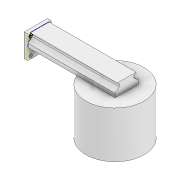
# Autodesk Inventor part: TopBracket
Saved by Autodesk Inventor 2021.1 (Build 251245010, 245A)
## iProperties
Created: 2023-07-02
Part Number: TopBracket
Material: ABS Plastic
Document SubType Name: Modeling
Designer: Drake
Density: 1.06 g/cm^3
Appearance: Smooth - White
Author: Drake
Autodesk Inventor part; units mm, degrees
ref_plane "YZ Plane" through (0, 0, 0) normal (1, 0, 0) x (0, 1, 0)
ref_plane "XZ Plane" through (0, 0, 0) normal (0, 1, 0) x (-1, 0, 0)
sketch "Sketch1" plane through (0, 0, 0) normal (1, 0, 0) x (0, 1, 0)
  line L0 (-20, 20) -> (20, 20)
  line L1 (20, 20) -> (20, -20)
  line L2 (20, -20) -> (-20, -20)
  line L3 (-20, -20) -> (-20, 20)
  line L4 (-20, 20) -> (20, -20) construction
  line L5 (20, 20) -> (-20, -20) construction
  point P0 (0, 0)
  dimension "d0" = 40
  dimension "d1" = 40
  constraints: 12 end point, 2 midpoint, 2 parallel, 1 horizontal, 1 perpendicular
  measures "d0" distance of L1.end L2.end
  measures "d1" distance of L0.end L1.end
extrude "Extrusion1" add sketch "Sketch1" along normal mid plane 6
sketch "Sketch2" plane through (3, 0, 0) normal (1, 0, 0) x (0, 0, -1)
  line L0 (20, 20) -> (-20, 20) projected
  line L1 (-20, 20) -> (-15, 20)
  line L2 (-15, 20) -> (-15, 15)
  line L3 (-15, 15) -> (-20, 15)
  line L4 (-20, 20) -> (-20, -20) projected
  circle A0 centre (-15, 15) radius 3
  point P0 (0, 0)
  dimension "d4" = 5
  dimension "d5" = 5
  dimension "d6" = 6
  constraints: 6 end point, 2 perpendicular, 2 point on line, 1 centre point, 1 coincident
  measures "d4" distance of L0.end L1.end
  measures "d5" distance of L1.end L2.end
  measures "d6" diameter of A0
extrude "Extrusion2" cut sketch "Sketch2" against normal blind 6 contours A0 L3 L2 | L2 L3 A0
mirror "Mirror1" about plane through (0, 0, 0) normal (0, 0, 1) of "Extrusion2"
mirror "Mirror2" about plane through (0, 0, 0) normal (0, 1, 0) of "Extrusion2", "Mirror1"
ref_plane "Work Plane4" through (0, 0, 20) normal (0, 0, -1) x (1, 0, 0)
ref_plane "Work Plane3" through (0, 0, 0) normal (0, 0, -1) x (1, 0, 0)
sketch "Sketch3" plane through (0, 0, 20) normal (0, 0, -1) x (1, 0, 0)
  line L0 (3, -20) -> (3, 20) projected
  line L1 (3, 0) -> (3, -15)
  line L2 (3, -15) -> (153, -15) construction
  line L3 (3, 0) -> (3, -7.5)
  point P0 (0, 0)
  dimension "d10" = 15
  dimension "bracketlength" = 150
  dimension "d12" = 7.5
  constraints: 6 end point, 2 midpoint, 1 horizontal, 1 point on line
  measures "d10" distance of L1.start L1.end
  measures "bracketlength" distance of L1.end L2.end
  measures "d12" distance of L1.start L3.end
sketch "Sketch4" plane through (3, 0, 0) normal (1, 0, 0) x (0, 0, -1)
  circle A0 centre (-15, 15) radius 3 projected
  circle A1 centre (15, 15) radius 3 projected
  circle A2 centre (-15, 15) radius 3 projected
  circle A3 centre (-15, 15) radius 3
  circle A4 centre (15, 15) radius 3
  line L0 (-20, 20) -> (20, 20) projected
  line L1 (-16.0857, 20) -> (-12.9984, 17.2346)
  line L2 (-17.7822, 15) -> (18, 15)
  circle A5 centre (15, 15) radius 3 projected
  line L3 (-16.0857, 10) -> (-12.9984, 12.7654)
  line L4 (0, 20) -> (0, 0)
  line L5 (-16.0857, 10) -> (-20, 6.4938)
  line L6 (-20, -20) -> (-20, 20) projected
  line L7 (-20, 6.4938) -> (-20, 0)
  circle A6 centre (15, 15) radius 3
  line L8 (16.0857, 20) -> (12.9984, 17.2346)
  line L9 (16.0857, 10) -> (12.9984, 12.7654)
  line L10 (16.0857, 10) -> (20, 6.4938)
  line L11 (20, 6.4938) -> (20, 0)
  line L12 (-16.0857, 20) -> (16.0857, 20)
  line L13 (-20, 0) -> (20, 0)
  constraints: 24 end point, 9 symmetric about line, 2 centre point, 2 coincident, 2 midpoint, 2 point on line, 1 collinear, 1 concentric, 1 horizontal, 1 horizontal alignment, 1 parallel, 1 vertical, 6 other
extrude "Extrusion3" add sketch "Sketch4" along normal blind 150 contours L2 L4 L13 L6 L5 L3 A0 | A0 L1 L0 L4 L2 | L4 L0 L8 A1 L2 | L2 A1 L9 L10 L11 L13 L4
sketch "Sketch5" plane through (3, 0, -20) normal (0, -1, 0) x (1, 0, 0)
  line L0 (150, 0) -> (150, 40)
  line L1 (150, 40) -> (150, 50)
  line L2 (150, 50) -> (150, -10)
  line L3 (150, 3.9143) -> (150, 36.0857) projected
  line L4 (150, 20) -> (110, 20)
  circle A0 centre (130, 20) radius 50
  point P0 (-3, 20)
  dimension "d15" = 10
  dimension "d16" = 60
  dimension "d17" = 40
  dimension "panmotorholderdiam" = 100
  constraints: 8 end point, 2 midpoint, 2 point on line, 1 centre point, 1 horizontal
  measures "d15" distance of L0.end L1.end
  measures "d16" distance of L1.end L2.end
  measures "d17" distance of L4.start L4.end
  measures "panmotorholderdiam" diameter of A0
extrude "Extrusion4" add sketch "Sketch5" along normal blind 80
sketch "Sketch6" plane through (133, -80, 0) normal (0, -1, 0) x (1, 0, 0)
  circle A0 centre (0, 0) radius 46.5
  point P0 (-133, 0)
  dimension "d21" = 93
  constraints: 1 centre point
  measures "d21" diameter of A0
extrude "Extrusion5" cut sketch "Sketch6" against normal blind 70
ref_plane "Work Plane1" through (0, 0, 0) normal (0, 0, 1) x (1, 0, 0)
ref_plane "Work Plane2" through (0, 0, 0) normal (0, 0, -1) x (1, 0, 0)
body "Solid1"
